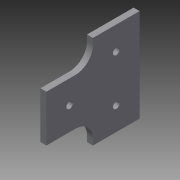
# Autodesk Inventor part: side holders
Saved by Autodesk Inventor 2015 (Build 190159000, 159)
## iProperties
Created: 2014-10-11
Part Number: side holders
Material: Generic
Document SubType Name: Modeling
Designer: jesse
Density: 1 g/cm^3
Appearance: Default
Author: jesse
Autodesk Inventor part; units mm, degrees
ref_plane "YZ Plane" through (0, 0, 0) normal (1, 0, 0) x (0, 1, 0)
ref_plane "XZ Plane" through (0, 0, 0) normal (0, 1, 0) x (-1, 0, 0)
ref_plane "XY Plane" through (0, 0, 0) normal (0, 0, 1) x (1, 0, 0)
sketch "Sketch1" plane through (0, 0, 0) normal (1, 0, 0) x (0, 1, 0)
  circle A0 centre (0, -38.1) radius 1.7907
  circle A1 centre (12.7, -12.7) radius 1.7907
  circle A2 centre (25.4, -38.1) radius 1.7907
  line L0 (-12.7, -50.8) -> (38.1, -50.8)
  line L1 (38.1, -25.4) -> (38.1, -50.8)
  line L2 (34.925, -25.4) -> (38.1, -25.4)
  arc A3 (25.4, -15.875) -> (34.925, -25.4) centre (34.925, -15.875) ccw
  line L3 (25.4, -15.875) -> (25.4, 0)
  line L4 (0, 0) -> (25.4, 0)
  line L5 (0, -15.875) -> (0, 0)
  arc A4 (-9.525, -25.4) -> (0, -15.875) centre (-9.525, -15.875) ccw
  line L6 (-9.525, -25.4) -> (-12.7, -25.4)
  line L7 (-12.7, -50.8) -> (-12.7, -25.4)
  point P0 (12.7, -50.8)
  constraints: 16 end point, 5 centre point, 4 point on circle
extrude "Extrusion1" add sketch "Sketch1" along normal blind 3.2512
body "Solid1"
